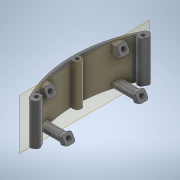
# Autodesk Inventor part: side_prot_stab
Saved by Autodesk Inventor 2020 (Build 240168000, 168)
## iProperties
Created: 2023-12-20
Part Number: side_prot_stab
Material: Пластик АБС
Document SubType Name: Modeling
Designer: denis
Density: 1.06 g/cm^3
Appearance: Гладкая — черная
Author: denis
Autodesk Inventor part; units mm, degrees
(part 1 of 3)
ref_plane "XZ Plane" through (0, 0, 0) normal (0, 1, 0) x (-1, 0, 0)
sketch "Эскиз1" plane through (0, 0, 0) normal (0, 1, 0) x (-1, 0, 0)
  arc A0 (93.050296, -48.648149) -> (93.050296, 48.648149) centre (0, 0) ccw
  line L0 (0, 0) -> (0, -105) construction
  line L1 (0, 0) -> (105, 0) construction
  line L2 (0, 0) -> (74.246212, -74.246212) construction
  line L3 (0, 0) -> (105, 0) construction
  arc A1 (47.06678, -85.957653) -> (85.957653, -47.06678) centre (0, 0) ccw construction
  line L4 (0, 0) -> (-74.246212, -74.246212) construction
  line L5 (73.892659, -46.315494) -> (46.315494, -73.892659)
  line L6 (76.013979, -34.294679) -> (34.294679, -76.013979)
  circle A2 centre (37.830213, -79.549513) radius 1.6
  circle A3 centre (79.549513, -37.830213) radius 1.6
  line L7 (37.830213, -79.549513) -> (79.549513, -37.830213) construction
  line L8 (87.179537, -38.389169) -> (83.085047, -34.294679)
  line L9 (38.389169, -87.179537) -> (34.294679, -83.085047)
  line L10 (88.270396, -49.379523) -> (85.206367, -46.315494)
  line L11 (49.379523, -88.270396) -> (46.315494, -85.206367)
  arc A4 (74.246212, -74.246212) -> (91.09999, -52.209117) centre (0, 0) ccw construction
  arc A5 (52.209117, -91.09999) -> (74.246212, -74.246212) centre (0, 0) ccw construction
  arc A6 (48.648149, -93.050296) -> (49.379523, -88.270396) centre (47.258202, -90.391716) ccw
  arc A7 (88.270396, -49.379523) -> (93.050296, -48.648149) centre (90.391716, -47.258202) ccw
  arc A8 (46.315494, -73.892659) -> (46.315494, -85.206367) centre (51.972348, -79.549513) ccw
  arc A9 (85.206367, -46.315494) -> (73.892659, -46.315494) centre (79.549513, -51.972348) ccw
  arc A10 (34.294679, -76.013979) -> (34.294679, -83.085047) centre (37.830213, -79.549513) ccw
  arc A11 (83.085047, -34.294679) -> (76.013979, -34.294679) centre (79.549513, -37.830213) ccw
  arc A12 (40.465243, -89.255611) -> (47.06678, -85.957653) centre (0, 0) ccw construction
  arc A13 (85.957653, -47.06678) -> (89.255611, -40.465243) centre (0, 0) ccw construction
  arc A14 (90.439454, -37.745267) -> (90.439454, 37.745267) centre (0, 0) ccw
  arc A15 (87.179537, -38.389169) -> (90.439454, -37.745267) centre (88.593751, -36.974956) ccw
  arc A16 (37.745267, -90.439454) -> (38.389169, -87.179537) centre (36.974956, -88.593751) ccw
  arc A17 (38.389169, 87.179537) -> (37.745267, 90.439454) centre (36.974956, 88.593751) ccw construction
  arc A18 (49.379523, 88.270396) -> (48.648149, 93.050296) centre (47.258202, 90.391716) ccw
  line L12 (49.379523, 88.270396) -> (46.315494, 85.206367)
  arc A19 (46.315494, 85.206367) -> (46.315494, 73.892659) centre (51.972348, 79.549513) ccw
  line L13 (38.389169, 87.179537) -> (34.294679, 83.085047) construction
  arc A20 (34.294679, 83.085047) -> (34.294679, 76.013979) centre (37.830213, 79.549513) ccw construction
  line L14 (34.294679, 76.013979) -> (76.013979, 34.294679) construction
  line L15 (46.315494, 73.892659) -> (73.892659, 46.315494)
  arc A21 (76.013979, 34.294679) -> (83.085047, 34.294679) centre (79.549513, 37.830213) ccw
  circle A22 centre (37.830213, 79.549513) radius 1.6
  circle A23 centre (79.549513, 37.830213) radius 1.6
  line L16 (87.179537, 38.389169) -> (83.085047, 34.294679)
  arc A24 (90.439454, 37.745267) -> (87.179537, 38.389169) centre (88.593751, 36.974956) ccw
  arc A25 (93.050296, 48.648149) -> (88.270396, 49.379523) centre (90.391716, 47.258202) ccw
  line L17 (88.270396, 49.379523) -> (85.206367, 46.315494)
  arc A26 (73.892659, 46.315494) -> (85.206367, 46.315494) centre (79.549513, 51.972348) ccw
  arc A27 (-87.179537, 38.389169) -> (-90.439454, 37.745267) centre (-88.593751, 36.974956) ccw
  arc A28 (-88.270396, 49.379523) -> (-93.050296, 48.648149) centre (-90.391716, 47.258202) ccw
  line L18 (-88.270396, 49.379523) -> (-85.206367, 46.315494)
  arc A29 (-85.206367, 46.315494) -> (-73.892659, 46.315494) centre (-79.549513, 51.972348) ccw
  line L19 (-87.179537, 38.389169) -> (-83.085047, 34.294679)
  arc A30 (-83.085047, 34.294679) -> (-76.013979, 34.294679) centre (-79.549513, 37.830213) ccw
  line L20 (-76.013979, 34.294679) -> (-34.294679, 76.013979) construction
  line L21 (-73.892659, 46.315494) -> (-46.315494, 73.892659)
  arc A31 (-34.294679, 76.013979) -> (-34.294679, 83.085047) centre (-37.830213, 79.549513) ccw construction
  circle A32 centre (-79.549513, 37.830213) radius 1.6
  circle A33 centre (-37.830213, 79.549513) radius 1.6
  line L22 (-38.389169, 87.179537) -> (-34.294679, 83.085047) construction
  arc A34 (-37.745267, 90.439454) -> (-38.389169, 87.179537) centre (-36.974956, 88.593751) ccw construction
  arc A35 (-48.648149, 93.050296) -> (-49.379523, 88.270396) centre (-47.258202, 90.391716) ccw
  line L23 (-49.379523, 88.270396) -> (-46.315494, 85.206367)
  arc A36 (-46.315494, 73.892659) -> (-46.315494, 85.206367) centre (-51.972348, 79.549513) ccw
  arc A37 (-38.389169, -87.179537) -> (-37.745267, -90.439454) centre (-36.974956, -88.593751) ccw
  arc A38 (-49.379523, -88.270396) -> (-48.648149, -93.050296) centre (-47.258202, -90.391716) ccw
  line L24 (-49.379523, -88.270396) -> (-46.315494, -85.206367)
  arc A39 (-46.315494, -85.206367) -> (-46.315494, -73.892659) centre (-51.972348, -79.549513) ccw
  line L25 (-38.389169, -87.179537) -> (-34.294679, -83.085047)
  arc A40 (-34.294679, -83.085047) -> (-34.294679, -76.013979) centre (-37.830213, -79.549513) ccw
  line L26 (-34.294679, -76.013979) -> (-76.013979, -34.294679)
  line L27 (-46.315494, -73.892659) -> (-73.892659, -46.315494)
  arc A41 (-76.013979, -34.294679) -> (-83.085047, -34.294679) centre (-79.549513, -37.830213) ccw
  circle A42 centre (-37.830213, -79.549513) radius 1.6
  circle A43 centre (-79.549513, -37.830213) radius 1.6
  line L28 (-87.179537, -38.389169) -> (-83.085047, -34.294679)
  arc A44 (-90.439454, -37.745267) -> (-87.179537, -38.389169) centre (-88.593751, -36.974956) ccw
  arc A45 (-93.050296, -48.648149) -> (-88.270396, -49.379523) centre (-90.391716, -47.258202) ccw
  line L29 (-88.270396, -49.379523) -> (-85.206367, -46.315494)
  arc A46 (-73.892659, -46.315494) -> (-85.206367, -46.315494) centre (-79.549513, -51.972348) ccw
  arc A47 (0, 67.941027) -> (23.782532, 76.596871) centre (0, 104.941027) ccw construction
  arc A48 (-23.782532, 76.596871) -> (0, 67.941027) centre (0, 104.941027) ccw construction
  line L30 (-23.782532, 76.596871) -> (-29.181616, 81.127042) construction
  arc A49 (-28.545172, 71.457103) -> (5.541335, 61.291358) centre (0, 104.941027) ccw construction
  arc A50 (5.541335, 61.291358) -> (28.545172, 71.457103) centre (0, 104.941027) ccw construction
  line L31 (23.782532, 76.596871) -> (26.803217, 79.131416) construction
  line L32 (-34.149097, 76.159561) -> (-28.545172, 71.457103) construction
  line L33 (31.223246, 73.704372) -> (28.545172, 71.457103) construction
  line L34 (26.803217, 79.131416) -> (23.782532, 76.596871) construction
  line L35 (30.759145, 79.549513) -> (31.448305, 78.860353) construction
  line L36 (31.223246, 73.704372) -> (28.545172, 71.457103) construction
  line L37 (-28.545172, 71.457103) -> (-34.149097, 76.159561) construction
  line L38 (-23.782532, 76.596871) -> (-29.181616, 81.127042) construction
  line L39 (-29.181616, 81.127042) -> (-34.149097, 76.159561) construction
  arc A51 (31.223246, 73.704372) -> (26.646177, 78.99965) centre (28.973431, 76.385479) ccw construction
  arc A52 (-26.646177, 78.99965) -> (-31.223246, 73.704372) centre (-28.973431, 76.385479) ccw construction
  arc A53 (-24.841986, 61.889251) -> (-25.418693, 62.824241) centre (-28.115423, 60.51553) ccw
  line L40 (-24.841986, 61.889251) -> (-23.83128, 59.480842)
  line L41 (-43.035533, 94.165467) -> (-18.380184, 65.366371)
  arc A54 (-0.616138, 59.304458) -> (0.616138, 59.304458) centre (0, 61.207186) ccw
  line L42 (-2.671978, 59.970176) -> (-4.5, 60.562123) construction
  arc A55 (-2.515557, 60.080545) -> (-2.671978, 59.970176) centre (0, 56.349329) ccw construction
  line L43 (-15.158499, 56.590699) -> (-21.004883, 57.332824)
  arc A56 (-14.511894, 56.446301) -> (-15.158499, 56.590699) centre (-15.605539, 53.068959) ccw
  line L44 (-17.477038, 64.764325) -> (-0.616138, 59.304458)
  line L45 (-14.511894, 56.446301) -> (-0.616138, 51.946601)
  arc A57 (44.027132, 95.32372) -> (43.576979, 95.530345) centre (0, 0) ccw construction
  circle A58 centre (20.557843, 60.854564) radius 1.55
  arc A59 (-34.190883, 73.070746) -> (-37.124381, 73.184277) centre (-35.710168, 71.770063) ccw
  line L46 (-34.190883, 73.070746) -> (-27.055798, 64.736489) construction
  line L47 (-25.418693, 62.824241) -> (-34.190883, 73.070746)
  arc A60 (-23.83128, 59.480842) -> (-21.004883, 57.332824) centre (-20.557843, 60.854564) ccw
  arc A61 (-18.380184, 65.366371) -> (-17.477038, 64.764325) centre (-16.8609, 66.667053) ccw
  circle A62 centre (-20.557843, 60.854564) radius 1.55
  arc A63 (15.158499, 56.590699) -> (14.511894, 56.446301) centre (15.605539, 53.068959) ccw
  line L48 (15.158499, 56.590699) -> (21.004883, 57.332824)
  arc A64 (25.418693, 62.824241) -> (24.841986, 61.889251) centre (28.115423, 60.51553) ccw
  line L49 (24.841986, 61.889251) -> (23.83128, 59.480842)
  arc A65 (21.004883, 57.332824) -> (23.83128, 59.480842) centre (20.557843, 60.854564) ccw
  line L50 (25.418693, 62.824241) -> (34.190883, 73.070746)
  arc A66 (37.124381, 73.184277) -> (34.190883, 73.070746) centre (35.710168, 71.770063) ccw
  line L51 (14.511894, 56.446301) -> (0.616138, 51.946601)
  arc A67 (17.477038, 64.764325) -> (18.380184, 65.366371) centre (16.8609, 66.667053) ccw
  line L52 (17.477038, 64.764325) -> (0.616138, 59.304458)
  line L53 (-37.124381, 73.184277) -> (-76.013979, 34.294679)
  line L54 (37.124381, 73.184277) -> (76.013979, 34.294679)
  arc A68 (-45.41996, 94.667984) -> (-48.648149, 93.050296) centre (0, 0) ccw
  arc A69 (-43.035533, 94.165467) -> (-45.41996, 94.667984) centre (-44.554817, 92.864785) ccw
  arc A70 (-0.616138, 51.946601) -> (0.616138, 51.946601) centre (0, 53.849329) ccw
  arc A71 (-48.648149, 93.050296) -> (-93.050296, 48.648149) centre (0, 0) ccw construction
  line L55 (43.035533, 94.165467) -> (18.380184, 65.366371)
  arc A72 (48.648149, 93.050296) -> (45.41996, 94.667984) centre (0, 0) ccw
  arc A73 (45.41996, 94.667984) -> (43.035533, 94.165467) centre (44.554817, 92.864785) ccw
  arc A74 (93.050296, 48.648149) -> (-44.027132, 95.32372) centre (0, 0) ccw construction
  arc A75 (-93.050296, -48.648149) -> (-48.648149, -93.050296) centre (0, 0) ccw construction
  arc A76 (-93.050296, 48.648149) -> (-93.050296, -48.648149) centre (0, 0) ccw
  arc A77 (-90.439454, -37.745267) -> (-37.745267, -90.439454) centre (0, 0) ccw construction
  arc A78 (-90.439454, 37.745267) -> (-90.439454, -37.745267) centre (0, 0) ccw
  arc A79 (90.439454, 37.745267) -> (-90.439454, 37.745267) centre (0, 0) ccw construction
  arc A80 (-37.745267, -90.439454) -> (37.745267, -90.439454) centre (0, 0) ccw
  arc A81 (-48.648149, -93.050296) -> (48.648149, -93.050296) centre (0, 0) ccw
  circle A82 centre (0, 55.599329) radius 1.75
  point P0 (60.104076, -60.104076)
  point P1 (55.154329, -55.154329)
  point P2 (78.135299, -39.244426)
  point P3 (39.244426, -78.135299)
  point P4 (52.209117, 91.09999)
  point P5 (39.244426, 78.135299)
  point P6 (47.06678, 85.957653)
  point P7 (55.154329, 55.154329)
  point P8 (60.104076, 60.104076)
  point P9 (91.09999, 52.209117)
  point P10 (78.135299, 39.244426)
  point P11 (85.957653, 47.06678)
  point P12 (-91.09999, 52.209117)
  point P13 (-78.135299, 39.244426)
  point P14 (-85.957653, 47.06678)
  point P15 (-55.154329, 55.154329)
  point P16 (-60.104076, 60.104076)
  point P17 (-52.209117, 91.09999)
  point P18 (-39.244426, 78.135299)
  point P19 (-47.06678, 85.957653)
  point P20 (-52.209117, -91.09999)
  point P21 (-39.244426, -78.135299)
  point P22 (-47.06678, -85.957653)
  point P23 (-55.154329, -55.154329)
  point P24 (-60.104076, -60.104076)
  point P25 (-91.09999, -52.209117)
  point P26 (-78.135299, -39.244426)
  point P27 (-85.957653, -47.06678)
  point P28 (-28.545172, 71.457103)
  point P29 (-39.282973, 89.782226)
  point P30 (0, 95.32372)
  point P31 (0, 66.207186)
  point P32 (-44.027132, 95.32372)
  point P33 (0, 59.207186)
  point P34 (44.554817, 92.864785)
  point P35 (-42.426407, 67.882251)
  point P36 (-22.705861, 58.028168)
  point P37 (-21.49571, 59.620504)
  dimension "d1" = 45
  dimension "d3" = 7
  dimension "d5" = 20
  dimension "d9" = 7
  dimension "d10" = 3.2
  dimension "d14" = 59
  dimension "d15" = 83
  dimension "d17" = 69
  dimension "d19" = 55
  dimension "d20" = 3
  dimension "d21" = 8
  dimension "d22" = 5
  dimension "d23" = 2
  dimension "d26" = 360
  dimension "d39" = 7
  dimension "d44" = 120
  dimension "d45" = 3.55
  dimension "d46" = 2
  dimension "d47" = 2.61189
  dimension "d48" = 2
  dimension "d49" = 105
  dimension "d50" = 2
  dimension "d54" = 3.5
  dimension "d55" = 2
  constraints: 165 point on circle, 112 end point, 83 centre point, 38 point on line, 27 tangent, 23 symmetric about line, 8 midpoint, 6 equal radius, 4 coincident, 4 collinear, 4 parallel, 3 horizontal, 2 vertical, 1 equal length, 1 perpendicular, 234 other
  measures "d1" angle of L2 L3
  measures "d3" radial gap between concentric circles of A0 A1
  measures "d5" distance from line of L5 L2.end
  measures "d9" distance between parallel lines of L5 L6
  measures "d10" diameter of A2
  measures "d14" distance of L7.end L7.start
  measures "d15" distance from line of point (0, 0) L7
  measures "d17" distance between parallel lines of L8 L9
  measures "d19" distance between parallel lines of L11 L10
  measures "d20" radius of A6
  measures "d21" radius of A8
  measures "d22" radius of A10
  measures "d23" radius of A15
  measures "d39" distance of point (0, 66.207) point (0, 59.207)
  measures "d44" angle of L40 L43
  measures "d45" radius of A53
  measures "d46" distance of point (-22.706, 58.028) point (-21.496, 59.621)
  measures "d47" distance of L40.start L40.end
  measures "d48" radius of A69
  measures "d49" radius of A68
  measures "d50" radius of A70
  measures "d54" diameter of A82
extrude "outer" add sketch "Эскиз1" along normal blind 2 contours A7 L10 A9 L5 A8 L11 A6 A81 A38 L24 A39 L27 A46 L29 A45 A76 A28 L18 A29 L21 A36 L23 A35 A68 A69 L41 A61 L44 A54 L52 A67 L55 A73 A72 A18 L12 A19 L15 A26 L17 A25 A0 | A82
sketch "Эскиз2" plane through (0, 2, 0) normal (0, 1, 0) x (1, 0, 0)
  arc A0 (-46.315494, -85.206367) -> (-46.315494, -73.892659) centre (-51.972348, -79.549513) ccw construction
  line L0 (-46.315494, -85.206367) -> (-49.379523, -88.270396) construction
  arc A1 (-49.379523, -88.270396) -> (-48.648149, -93.050296) centre (-47.258202, -90.391716) ccw construction
  arc A2 (-48.648149, -93.050296) -> (-45.41996, -94.667984) centre (0, 0) ccw construction
  arc A3 (-45.41996, -94.667984) -> (-43.035533, -94.165467) centre (-44.554817, -92.864785) ccw construction
  line L1 (-43.035533, -94.165467) -> (-18.380184, -65.366371) construction
  arc A4 (-17.477038, -64.764325) -> (-18.380184, -65.366371) centre (-16.8609, -66.667053) ccw construction
  line L2 (-17.477038, -64.764325) -> (-0.616138, -59.304458) construction
  arc A5 (0.616138, -59.304458) -> (-0.616138, -59.304458) centre (0, -61.207186) ccw construction
  line L3 (0.616138, -59.304458) -> (17.477038, -64.764325) construction
  arc A6 (18.380184, -65.366371) -> (17.477038, -64.764325) centre (16.8609, -66.667053) ccw construction
  line L4 (18.380184, -65.366371) -> (43.035533, -94.165467) construction
  arc A7 (43.035533, -94.165467) -> (45.41996, -94.667984) centre (44.554817, -92.864785) ccw construction
  arc A8 (45.41996, -94.667984) -> (48.648149, -93.050296) centre (0, 0) ccw construction
  arc A9 (48.648149, -93.050296) -> (49.379523, -88.270396) centre (47.258202, -90.391716) ccw construction
  line L5 (49.379523, -88.270396) -> (46.315494, -85.206367) construction
  arc A10 (46.315494, -73.892659) -> (46.315494, -85.206367) centre (51.972348, -79.549513) ccw construction
  line L6 (46.315494, -73.892659) -> (73.892659, -46.315494) construction
  arc A11 (85.206367, -46.315494) -> (73.892659, -46.315494) centre (79.549513, -51.972348) ccw construction
  line L7 (85.206367, -46.315494) -> (88.270396, -49.379523) construction
  arc A12 (88.270396, -49.379523) -> (93.050296, -48.648149) centre (90.391716, -47.258202) ccw construction
  arc A13 (93.050296, -48.648149) -> (93.050296, 48.648149) centre (0, 0) ccw construction
  arc A14 (93.050296, 48.648149) -> (88.270396, 49.379523) centre (90.391716, 47.258202) ccw construction
  line L8 (88.270396, 49.379523) -> (85.206367, 46.315494) construction
  arc A15 (73.892659, 46.315494) -> (85.206367, 46.315494) centre (79.549513, 51.972348) ccw construction
  line L9 (73.892659, 46.315494) -> (46.315494, 73.892659) construction
  arc A16 (46.315494, 85.206367) -> (46.315494, 73.892659) centre (51.972348, 79.549513) ccw construction
  line L10 (46.315494, 85.206367) -> (49.379523, 88.270396) construction
  arc A17 (49.379523, 88.270396) -> (48.648149, 93.050296) centre (47.258202, 90.391716) ccw construction
  arc A18 (48.648149, 93.050296) -> (-48.648149, 93.050296) centre (0, 0) ccw construction
  arc A19 (-48.648149, 93.050296) -> (-49.379523, 88.270396) centre (-47.258202, 90.391716) ccw construction
  line L11 (-49.379523, 88.270396) -> (-46.315494, 85.206367) construction
  arc A20 (-46.315494, 73.892659) -> (-46.315494, 85.206367) centre (-51.972348, 79.549513) ccw construction
  line L12 (-46.315494, 73.892659) -> (-73.892659, 46.315494) construction
  arc A21 (-85.206367, 46.315494) -> (-73.892659, 46.315494) centre (-79.549513, 51.972348) ccw construction
  line L13 (-85.206367, 46.315494) -> (-88.270396, 49.379523) construction
  arc A22 (-88.270396, 49.379523) -> (-93.050296, 48.648149) centre (-90.391716, 47.258202) ccw construction
  arc A23 (-93.050296, 48.648149) -> (-93.050296, -48.648149) centre (0, 0) ccw construction
  arc A24 (-93.050296, -48.648149) -> (-88.270396, -49.379523) centre (-90.391716, -47.258202) ccw construction
  line L14 (-88.270396, -49.379523) -> (-85.206367, -46.315494) construction
  arc A25 (-73.892659, -46.315494) -> (-85.206367, -46.315494) centre (-79.549513, -51.972348) ccw construction
  line L15 (-73.892659, -46.315494) -> (-46.315494, -73.892659) construction
  circle A26 centre (-37.830213, 79.549513) radius 1.6 construction
  circle A27 centre (-79.549513, 37.830213) radius 1.6 construction
  circle A28 centre (-79.549513, -37.830213) radius 1.6 construction
  circle A29 centre (79.549513, -37.830213) radius 1.6 construction
  circle A30 centre (37.830213, 79.549513) radius 1.6 construction
  circle A31 centre (79.549513, 37.830213) radius 1.6 construction
  circle A32 centre (-20.557843, -60.854564) radius 1.55 construction
  circle A33 centre (20.557843, -60.854564) radius 1.55 construction
  circle A34 centre (37.830213, -79.549513) radius 1.6 construction
  circle A35 centre (-37.830213, -79.549513) radius 1.6 construction
  line L16 (-83.085047, -34.294679) -> (-87.179537, -38.389169) construction
  arc A36 (-90.439454, -37.745267) -> (-87.179537, -38.389169) centre (-88.593751, -36.974956) ccw construction
  arc A37 (-90.439454, 37.745267) -> (-90.439454, -37.745267) centre (0, 0) ccw construction
  arc A38 (-87.179537, 38.389169) -> (-90.439454, 37.745267) centre (-88.593751, 36.974956) ccw construction
  line L17 (-87.179537, 38.389169) -> (-83.085047, 34.294679) construction
  arc A39 (-83.085047, 34.294679) -> (-76.013979, 34.294679) centre (-79.549513, 37.830213) ccw construction
  line L18 (-76.013979, 34.294679) -> (-34.294679, 76.013979) construction
  arc A40 (-34.294679, 76.013979) -> (-34.294679, 83.085047) centre (-37.830213, 79.549513) ccw construction
  line L19 (-34.294679, 83.085047) -> (-38.389169, 87.179537) construction
  arc A41 (-37.745267, 90.439454) -> (-38.389169, 87.179537) centre (-36.974956, 88.593751) ccw construction
  arc A42 (37.745267, 90.439454) -> (-37.745267, 90.439454) centre (0, 0) ccw construction
  arc A43 (38.389169, 87.179537) -> (37.745267, 90.439454) centre (36.974956, 88.593751) ccw construction
  line L20 (38.389169, 87.179537) -> (34.294679, 83.085047) construction
  arc A44 (34.294679, 83.085047) -> (34.294679, 76.013979) centre (37.830213, 79.549513) ccw construction
  line L21 (34.294679, 76.013979) -> (76.013979, 34.294679) construction
  arc A45 (76.013979, 34.294679) -> (83.085047, 34.294679) centre (79.549513, 37.830213) ccw construction
  line L22 (83.085047, 34.294679) -> (87.179537, 38.389169) construction
  arc A46 (90.439454, 37.745267) -> (87.179537, 38.389169) centre (88.593751, 36.974956) ccw construction
  arc A47 (90.439454, -37.745267) -> (90.439454, 37.745267) centre (0, 0) ccw construction
  arc A48 (87.179537, -38.389169) -> (90.439454, -37.745267) centre (88.593751, -36.974956) ccw construction
  line L23 (87.179537, -38.389169) -> (83.085047, -34.294679) construction
  arc A49 (83.085047, -34.294679) -> (76.013979, -34.294679) centre (79.549513, -37.830213) ccw construction
  line L24 (76.013979, -34.294679) -> (37.124381, -73.184277) construction
  arc A50 (34.190883, -73.070746) -> (37.124381, -73.184277) centre (35.710168, -71.770063) ccw construction
  line L25 (34.190883, -73.070746) -> (25.418693, -62.824241) construction
  arc A51 (24.841986, -61.889251) -> (25.418693, -62.824241) centre (28.115423, -60.51553) ccw construction
  line L26 (24.841986, -61.889251) -> (23.83128, -59.480842) construction
  arc A52 (23.83128, -59.480842) -> (21.004883, -57.332824) centre (20.557843, -60.854564) ccw construction
  line L27 (21.004883, -57.332824) -> (15.158499, -56.590699) construction
  arc A53 (14.511894, -56.446301) -> (15.158499, -56.590699) centre (15.605539, -53.068959) ccw construction
  line L28 (14.511894, -56.446301) -> (0.616138, -51.946601) construction
  arc A54 (0.616138, -51.946601) -> (-0.616138, -51.946601) centre (0, -53.849329) ccw construction
  line L29 (-0.616138, -51.946601) -> (-14.511894, -56.446301) construction
  arc A55 (-15.158499, -56.590699) -> (-14.511894, -56.446301) centre (-15.605539, -53.068959) ccw construction
  line L30 (-15.158499, -56.590699) -> (-21.004883, -57.332824) construction
  arc A56 (-21.004883, -57.332824) -> (-23.83128, -59.480842) centre (-20.557843, -60.854564) ccw construction
  line L31 (-23.83128, -59.480842) -> (-24.841986, -61.889251) construction
  arc A57 (-25.418693, -62.824241) -> (-24.841986, -61.889251) centre (-28.115423, -60.51553) ccw construction
  line L32 (-25.418693, -62.824241) -> (-34.190883, -73.070746) construction
  arc A58 (-37.124381, -73.184277) -> (-34.190883, -73.070746) centre (-35.710168, -71.770063) ccw construction
  line L33 (-37.124381, -73.184277) -> (-76.013979, -34.294679) construction
  arc A59 (-76.013979, -34.294679) -> (-83.085047, -34.294679) centre (-79.549513, -37.830213) ccw construction
  line L34 (0, 0) -> (-74.246212, 74.246212) construction
  line L35 (0, 0) -> (-105, 0) construction
  line L36 (0, 0) -> (0, 105) construction
  line L37 (0, 0) -> (74.246212, 74.246212) construction
  line L38 (-46.669048, 63.63961) -> (-26.870058, 43.84062)
  line L39 (-63.63961, 46.669048) -> (-43.84062, 26.870058)
  line L40 (-67.882251, 42.426407) -> (-43.133514, 17.67767) construction
  line L41 (-41.012193, 26.870058) -> (-26.870058, 41.012193)
  line L42 (-43.134692, 17.676491) -> (-17.67767, 43.133514) construction
  circle A60 centre (-21.92031, 43.133514) radius 1.6
  circle A61 centre (-43.133514, 21.92031) radius 1.6
  line L43 (-33.941125, 33.941125) -> (-30.405592, 30.405592) construction
  arc A62 (-26.870058, 41.012193) -> (-26.870058, 43.84062) centre (-28.284271, 42.426407) ccw
  arc A63 (-43.84062, 26.870058) -> (-41.012193, 26.870058) centre (-42.426407, 28.284271) ccw
  line L44 (-67.882251, 42.426407) -> (-42.426407, 67.882251)
  line L45 (-43.133514, 21.92031) -> (-21.92031, 43.133514) construction
  line L46 (-63.63961, -46.669048) -> (-43.84062, -26.870058)
  line L47 (-42.426407, -67.882251) -> (-67.882251, -42.426407)
  line L48 (-46.669048, -63.63961) -> (-26.870058, -43.84062)
  line L49 (-26.870058, -41.012193) -> (-41.012193, -26.870058)
  arc A64 (-41.012193, -26.870058) -> (-43.84062, -26.870058) centre (-42.426407, -28.284271) ccw
  circle A65 centre (-43.133514, -21.92031) radius 1.6
  circle A66 centre (-21.92031, -43.133514) radius 1.6
  arc A67 (-26.870058, -43.84062) -> (-26.870058, -41.012193) centre (-28.284271, -42.426407) ccw
  line L50 (46.669048, -63.63961) -> (26.870058, -43.84062)
  line L51 (67.882251, -42.426407) -> (42.426407, -67.882251)
  line L52 (63.63961, -46.669048) -> (43.84062, -26.870058)
  line L53 (41.012193, -26.870058) -> (26.870058, -41.012193)
  arc A68 (26.870058, -41.012193) -> (26.870058, -43.84062) centre (28.284271, -42.426407) ccw
  circle A69 centre (21.92031, -43.133514) radius 1.6
  circle A70 centre (43.133514, -21.92031) radius 1.6
  arc A71 (43.84062, -26.870058) -> (41.012193, -26.870058) centre (42.426407, -28.284271) ccw
  line L54 (63.63961, 46.669048) -> (43.84062, 26.870058)
  line L55 (42.426407, 67.882251) -> (67.882251, 42.426407)
  line L56 (46.669048, 63.63961) -> (26.870058, 43.84062)
  line L57 (26.870058, 41.012193) -> (41.012193, 26.870058)
  arc A72 (41.012193, 26.870058) -> (43.84062, 26.870058) centre (42.426407, 28.284271) ccw
  circle A73 centre (43.133514, 21.92031) radius 1.6
  circle A74 centre (21.92031, 43.133514) radius 1.6
  arc A75 (26.870058, 43.84062) -> (26.870058, 41.012193) centre (28.284271, 42.426407) ccw
  line L58 (-21.92031, 43.133514) -> (21.92031, 43.133514) construction
  line L59 (-20.67767, 40.133514) -> (20.67767, 40.133514) construction
  line L60 (-20.67767, 46.133514) -> (20.67767, 46.133514) construction
  line L61 (42.426407, 67.882251) -> (14.225288, 39.681132) construction
  line L62 (67.882251, 42.426407) -> (40.318778, 14.862934) construction
  line L63 (43.134692, 17.676491) -> (16.615831, 44.195352) construction
  arc A76 (-21.669819, 47.125663) -> (-21.669819, 39.141365) centre (-21.92031, 43.133514) ccw construction
  line L64 (-42.426407, 67.882251) -> (-21.669819, 47.125663)
  arc A77 (-19.274559, 46.133514) -> (-21.669819, 47.125663) centre (-21.92031, 43.133514) ccw
  arc A78 (-21.669819, 39.141365) -> (-19.274559, 40.133514) centre (-21.92031, 43.133514) ccw
  arc A79 (-19.274559, 40.133514) -> (-19.274559, 46.133514) centre (-21.92031, 43.133514) ccw construction
  line L65 (-21.669819, 47.125663) -> (-17.67767, 43.133514) construction
  line L66 (-19.274559, 46.133514) -> (0, 46.133514)
  line L67 (-30.405592, 30.405592) -> (-21.669819, 39.141365)
  line L68 (-67.882251, 42.426407) -> (-47.125663, 21.669819)
  arc A80 (-47.125663, 21.669819) -> (-46.133514, 19.274559) centre (-43.133514, 21.92031) ccw
  arc A81 (-40.133514, 19.274559) -> (-39.141365, 21.669819) centre (-43.133514, 21.92031) ccw
  line L69 (-46.133514, 19.274559) -> (-46.133514, 0)
  line L70 (-30.405592, 30.405592) -> (-39.141365, 21.669819)
  line L71 (-19.274559, 40.133514) -> (0, 40.133514)
  line L72 (-40.133514, 19.274559) -> (-40.133514, 0)
  line L73 (-40.133514, -19.274559) -> (-40.133514, 0)
  line L74 (-46.133514, -19.274559) -> (-46.133514, 0)
  arc A82 (-46.133514, -19.274559) -> (-47.125663, -21.669819) centre (-43.133514, -21.92031) ccw
  line L75 (-67.882251, -42.426407) -> (-47.125663, -21.669819)
  arc A83 (-39.141365, -21.669819) -> (-40.133514, -19.274559) centre (-43.133514, -21.92031) ccw
  line L76 (-30.405592, -30.405592) -> (-39.141365, -21.669819)
  line L77 (-30.405592, -30.405592) -> (-21.669819, -39.141365)
  arc A84 (-19.274559, -40.133514) -> (-21.669819, -39.141365) centre (-21.92031, -43.133514) ccw
  line L78 (-19.274559, -40.133514) -> (0, -40.133514)
  line L79 (-19.274559, -46.133514) -> (0, -46.133514)
  arc A85 (-21.669819, -47.125663) -> (-19.274559, -46.133514) centre (-21.92031, -43.133514) ccw
  line L80 (-42.426407, -67.882251) -> (-21.669819, -47.125663)
  line L81 (19.274559, -40.133514) -> (0, -40.133514)
  line L82 (19.274559, -46.133514) -> (0, -46.133514)
  arc A86 (19.274559, -46.133514) -> (21.669819, -47.125663) centre (21.92031, -43.133514) ccw
  line L83 (42.426407, -67.882251) -> (21.669819, -47.125663)
  arc A87 (21.669819, -39.141365) -> (19.274559, -40.133514) centre (21.92031, -43.133514) ccw
  line L84 (30.405592, -30.405592) -> (21.669819, -39.141365)
  line L85 (30.405592, -30.405592) -> (39.141365, -21.669819)
  arc A88 (40.133514, -19.274559) -> (39.141365, -21.669819) centre (43.133514, -21.92031) ccw
  line L86 (40.133514, -19.274559) -> (40.133514, 0)
  line L87 (46.133514, -19.274559) -> (46.133514, 0)
  arc A89 (47.125663, -21.669819) -> (46.133514, -19.274559) centre (43.133514, -21.92031) ccw
  line L88 (67.882251, -42.426407) -> (47.125663, -21.669819)
  line L89 (40.133514, 19.274559) -> (40.133514, 0)
  line L90 (46.133514, 19.274559) -> (46.133514, 0)
  arc A90 (46.133514, 19.274559) -> (47.125663, 21.669819) centre (43.133514, 21.92031) ccw
  line L91 (67.882251, 42.426407) -> (47.125663, 21.669819)
  arc A91 (39.141365, 21.669819) -> (40.133514, 19.274559) centre (43.133514, 21.92031) ccw
  line L92 (30.405592, 30.405592) -> (39.141365, 21.669819)
  line L93 (30.405592, 30.405592) -> (21.669819, 39.141365)
  arc A92 (19.274559, 40.133514) -> (21.669819, 39.141365) centre (21.92031, 43.133514) ccw
  line L94 (19.274559, 40.133514) -> (0, 40.133514)
  line L95 (19.274559, 46.133514) -> (0, 46.133514)
  arc A93 (21.669819, 47.125663) -> (19.274559, 46.133514) centre (21.92031, 43.133514) ccw
  line L96 (42.426407, 67.882251) -> (21.669819, 47.125663)
  point P0 (-25.455844, 42.426407)
  point P1 (-32.173359, 32.173359)
  point P2 (-42.426407, -25.455844)
  point P3 (-33.941125, -33.941125)
  point P4 (25.455844, -42.426407)
  point P5 (33.941125, -33.941125)
  point P6 (42.426407, 25.455844)
  point P7 (33.941125, 33.941125)
  point P8 (-46.133514, -20.67767)
  point P9 (20.67767, -46.133514)
  point P10 (46.133514, 20.67767)
  point P11 (0, 46.133514)
  point P12 (-46.133514, 0)
  point P13 (0, -46.133514)
  point P14 (46.133514, 0)
  point P15 (0, 40.133514)
  point P16 (40.133514, 0)
  point P17 (0, -40.133514)
  point P18 (-40.133514, 0)
  dimension "d58" = 12
  dimension "d59" = 30
  dimension "d60" = 5
  dimension "d61" = 3.2
  dimension "d62" = 30
  dimension "d63" = 2
  dimension "d64" = 2
  dimension "d65" = 3
  dimension "d68" = 360
  dimension "d70" = 6
  dimension "d71" = 8
  dimension "d74" = 360
  constraints: 118 end point, 52 point on circle, 34 centre point, 28 point on line, 8 symmetric about line, 5 parallel, 4 midpoint, 4 tangent, 1 coincident, 1 collinear, 1 horizontal, 1 perpendicular, 216 other
  measures "d58" distance between parallel lines of L34 L38
  measures "d59" distance between parallel lines of L18 L41
  measures "d60" distance between parallel lines of L41 L42
  measures "d61" diameter of A60
  measures "d62" distance of L45.start L45.end
  measures "d63" radius of A62
  measures "d64" radius of A63
  measures "d65" distance between parallel lines of L42 L45
  measures "d70" distance between parallel lines of L59 L60
  measures "d71" diameter of A76
extrude "inner" add sketch "Эскиз2" against normal blind 2 contours L44 L64 A77 L66 L95 A93 L96 L55 L56 A75 L57 A72 L54 L91 A90 L90 L87 A89 L88 L51 L52 A71 L53 A68 L50 L83 A86 L82 L79 A85 L80 L47 L48 A67 L49 A64 L46 L75 A82 L74 L69 A80 L68 L39 A63 L41 A62 L38
sketch "Эскиз3" plane through (0, 2, 0) normal (0, 1, 0) x (1, 0, 0)
  line L0 (-40.133514, -19.274559) -> (-40.133514, 19.274559) construction
  line L1 (-67.882251, -42.426407) -> (-76.013979, -34.294679) construction
  arc A0 (-76.013979, -34.294679) -> (-83.085047, -34.294679) centre (-79.549513, -37.830213) ccw construction
  line L2 (-83.085047, -34.294679) -> (-87.179537, -38.389169) construction
  arc A1 (-90.439454, -37.745267) -> (-87.179537, -38.389169) centre (-88.593751, -36.974956) ccw construction
  arc A2 (-90.439454, 37.745267) -> (-90.439454, -37.745267) centre (0, 0) ccw construction
  arc A3 (-87.179537, 38.389169) -> (-90.439454, 37.745267) centre (-88.593751, 36.974956) ccw construction
  line L3 (-87.179537, 38.389169) -> (-83.085047, 34.294679) construction
  arc A4 (-83.085047, 34.294679) -> (-76.013979, 34.294679) centre (-79.549513, 37.830213) ccw construction
  line L4 (-76.013979, 34.294679) -> (-67.882251, 42.426407) construction
  line L5 (-67.882251, 42.426407) -> (-47.125663, 21.669819) construction
  arc A5 (-47.125663, 21.669819) -> (-46.133514, 19.274559) centre (-43.133514, 21.92031) ccw construction
  line L6 (-46.133514, 19.274559) -> (-46.133514, -19.274559) construction
  arc A6 (-46.133514, -19.274559) -> (-47.125663, -21.669819) centre (-43.133514, -21.92031) ccw construction
  line L7 (-47.125663, -21.669819) -> (-67.882251, -42.426407) construction
  line L8 (-63.63961, -46.669048) -> (-43.84062, -26.870058) construction
  arc A7 (-41.012193, -26.870058) -> (-43.84062, -26.870058) centre (-42.426407, -28.284271) ccw construction
  line L9 (-41.012193, -26.870058) -> (-26.870058, -41.012193) construction
  arc A8 (-26.870058, -43.84062) -> (-26.870058, -41.012193) centre (-28.284271, -42.426407) ccw construction
  line L10 (-26.870058, -43.84062) -> (-46.669048, -63.63961) construction
  line L11 (-46.669048, -63.63961) -> (-63.63961, -46.669048) construction
  line L12 (-42.426407, -67.882251) -> (-21.669819, -47.125663) construction
  arc A9 (-21.669819, -47.125663) -> (-19.274559, -46.133514) centre (-21.92031, -43.133514) ccw construction
  line L13 (-19.274559, -46.133514) -> (19.274559, -46.133514) construction
  arc A10 (19.274559, -46.133514) -> (21.669819, -47.125663) centre (21.92031, -43.133514) ccw construction
  line L14 (21.669819, -47.125663) -> (42.426407, -67.882251) construction
  line L15 (42.426407, -67.882251) -> (37.124381, -73.184277) construction
  arc A11 (34.190883, -73.070746) -> (37.124381, -73.184277) centre (35.710168, -71.770063) ccw construction
  line L16 (34.190883, -73.070746) -> (25.418693, -62.824241) construction
  arc A12 (24.841986, -61.889251) -> (25.418693, -62.824241) centre (28.115423, -60.51553) ccw construction
  line L17 (24.841986, -61.889251) -> (23.83128, -59.480842) construction
  arc A13 (23.83128, -59.480842) -> (21.004883, -57.332824) centre (20.557843, -60.854564) ccw construction
  line L18 (21.004883, -57.332824) -> (15.158499, -56.590699) construction
  arc A14 (14.511894, -56.446301) -> (15.158499, -56.590699) centre (15.605539, -53.068959) ccw construction
  line L19 (14.511894, -56.446301) -> (0.616138, -51.946601) construction
  arc A15 (0.616138, -51.946601) -> (-0.616138, -51.946601) centre (0, -53.849329) ccw construction
  line L20 (-0.616138, -51.946601) -> (-14.511894, -56.446301) construction
  arc A16 (-15.158499, -56.590699) -> (-14.511894, -56.446301) centre (-15.605539, -53.068959) ccw construction
  line L21 (-15.158499, -56.590699) -> (-21.004883, -57.332824) construction
  arc A17 (-21.004883, -57.332824) -> (-23.83128, -59.480842) centre (-20.557843, -60.854564) ccw construction
  line L22 (-23.83128, -59.480842) -> (-24.841986, -61.889251) construction
  arc A18 (-25.418693, -62.824241) -> (-24.841986, -61.889251) centre (-28.115423, -60.51553) ccw construction
  line L23 (-25.418693, -62.824241) -> (-34.190883, -73.070746) construction
  arc A19 (-37.124381, -73.184277) -> (-34.190883, -73.070746) centre (-35.710168, -71.770063) ccw construction
  line L24 (-37.124381, -73.184277) -> (-42.426407, -67.882251) construction
  line L25 (46.669048, -63.63961) -> (26.870058, -43.84062) construction
  arc A20 (26.870058, -41.012193) -> (26.870058, -43.84062) centre (28.284271, -42.426407) ccw construction
  line L26 (26.870058, -41.012193) -> (41.012193, -26.870058) construction
  arc A21 (43.84062, -26.870058) -> (41.012193, -26.870058) centre (42.426407, -28.284271) ccw construction
  line L27 (43.84062, -26.870058) -> (63.63961, -46.669048) construction
  line L28 (63.63961, -46.669048) -> (46.669048, -63.63961) construction
  line L29 (67.882251, -42.426407) -> (47.125663, -21.669819) construction
  arc A22 (47.125663, -21.669819) -> (46.133514, -19.274559) centre (43.133514, -21.92031) ccw construction
  line L30 (46.133514, -19.274559) -> (46.133514, 19.274559) construction
  arc A23 (46.133514, 19.274559) -> (47.125663, 21.669819) centre (43.133514, 21.92031) ccw construction
  line L31 (47.125663, 21.669819) -> (67.882251, 42.426407) construction
  line L32 (67.882251, 42.426407) -> (76.013979, 34.294679) construction
  arc A24 (76.013979, 34.294679) -> (83.085047, 34.294679) centre (79.549513, 37.830213) ccw construction
  line L33 (83.085047, 34.294679) -> (87.179537, 38.389169) construction
  arc A25 (90.439454, 37.745267) -> (87.179537, 38.389169) centre (88.593751, 36.974956) ccw construction
  arc A26 (90.439454, -37.745267) -> (90.439454, 37.745267) centre (0, 0) ccw construction
  arc A27 (87.179537, -38.389169) -> (90.439454, -37.745267) centre (88.593751, -36.974956) ccw construction
  line L34 (87.179537, -38.389169) -> (83.085047, -34.294679) construction
  arc A28 (83.085047, -34.294679) -> (76.013979, -34.294679) centre (79.549513, -37.830213) ccw construction
  line L35 (76.013979, -34.294679) -> (67.882251, -42.426407) construction
  line L36 (63.63961, 46.669048) -> (43.84062, 26.870058) construction
  arc A29 (41.012193, 26.870058) -> (43.84062, 26.870058) centre (42.426407, 28.284271) ccw construction
  line L37 (41.012193, 26.870058) -> (26.870058, 41.012193) construction
  arc A30 (26.870058, 43.84062) -> (26.870058, 41.012193) centre (28.284271, 42.426407) ccw construction
  line L38 (26.870058, 43.84062) -> (46.669048, 63.63961) construction
  line L39 (46.669048, 63.63961) -> (63.63961, 46.669048) construction
  line L40 (42.426407, 67.882251) -> (21.669819, 47.125663) construction
  arc A31 (21.669819, 47.125663) -> (19.274559, 46.133514) centre (21.92031, 43.133514) ccw construction
  line L41 (19.274559, 46.133514) -> (-19.274559, 46.133514) construction
  arc A32 (-19.274559, 46.133514) -> (-21.669819, 47.125663) centre (-21.92031, 43.133514) ccw construction
  line L42 (-21.669819, 47.125663) -> (-42.426407, 67.882251) construction
  line L43 (-42.426407, 67.882251) -> (-34.294679, 76.013979) construction
  arc A33 (-34.294679, 76.013979) -> (-34.294679, 83.085047) centre (-37.830213, 79.549513) ccw construction
  line L44 (-34.294679, 83.085047) -> (-38.389169, 87.179537) construction
  arc A34 (-37.745267, 90.439454) -> (-38.389169, 87.179537) centre (-36.974956, 88.593751) ccw construction
  arc A35 (37.745267, 90.439454) -> (-37.745267, 90.439454) centre (0, 0) ccw construction
  arc A36 (38.389169, 87.179537) -> (37.745267, 90.439454) centre (36.974956, 88.593751) ccw construction
  line L45 (38.389169, 87.179537) -> (34.294679, 83.085047) construction
  arc A37 (34.294679, 83.085047) -> (34.294679, 76.013979) centre (37.830213, 79.549513) ccw construction
  line L46 (34.294679, 76.013979) -> (42.426407, 67.882251) construction
  line L47 (-19.274559, 40.133514) -> (19.274559, 40.133514) construction
  arc A38 (19.274559, 40.133514) -> (21.669819, 39.141365) centre (21.92031, 43.133514) ccw construction
  line L48 (21.669819, 39.141365) -> (39.141365, 21.669819) construction
  arc A39 (39.141365, 21.669819) -> (40.133514, 19.274559) centre (43.133514, 21.92031) ccw construction
  line L49 (40.133514, 19.274559) -> (40.133514, -19.274559) construction
  arc A40 (40.133514, -19.274559) -> (39.141365, -21.669819) centre (43.133514, -21.92031) ccw construction
  line L50 (39.141365, -21.669819) -> (21.669819, -39.141365) construction
  arc A41 (21.669819, -39.141365) -> (19.274559, -40.133514) centre (21.92031, -43.133514) ccw construction
  line L51 (19.274559, -40.133514) -> (-19.274559, -40.133514) construction
  arc A42 (-19.274559, -40.133514) -> (-21.669819, -39.141365) centre (-21.92031, -43.133514) ccw construction
  line L52 (-21.669819, -39.141365) -> (-39.141365, -21.669819) construction
  arc A43 (-39.141365, -21.669819) -> (-40.133514, -19.274559) centre (-43.133514, -21.92031) ccw construction
  line L53 (-40.133514, -19.274559) -> (-40.133514, 19.274559) construction
  arc A44 (-40.133514, 19.274559) -> (-39.141365, 21.669819) centre (-43.133514, 21.92031) ccw construction
  line L54 (-39.141365, 21.669819) -> (-21.669819, 39.141365) construction
  arc A45 (-21.669819, 39.141365) -> (-19.274559, 40.133514) centre (-21.92031, 43.133514) ccw construction
  circle A46 centre (43.133514, 21.92031) radius 1.6 construction
  circle A47 centre (21.92031, -43.133514) radius 1.6 construction
  circle A48 centre (-21.92031, -43.133514) radius 1.6 construction
  circle A49 centre (-43.133514, -21.92031) radius 1.6 construction
  circle A50 centre (-43.133514, 21.92031) radius 1.6 construction
  circle A51 centre (-21.92031, 43.133514) radius 1.6 construction
  circle A52 centre (43.133514, -21.92031) radius 1.6 construction
  circle A53 centre (21.92031, 43.133514) radius 1.6 construction
  arc A54 (-88.270396, 49.379523) -> (-93.050296, 48.648149) centre (-90.391716, 47.258202) ccw construction
  arc A55 (-93.050296, 48.648149) -> (-93.050296, -48.648149) centre (0, 0) ccw construction
  arc A56 (-93.050296, -48.648149) -> (-88.270396, -49.379523) centre (-90.391716, -47.258202) ccw construction
  line L55 (-88.270396, -49.379523) -> (-85.206367, -46.315494) construction
  arc A57 (-73.892659, -46.315494) -> (-85.206367, -46.315494) centre (-79.549513, -51.972348) ccw construction
  line L56 (-73.892659, -46.315494) -> (-46.315494, -73.892659) construction
  arc A58 (-46.315494, -85.206367) -> (-46.315494, -73.892659) centre (-51.972348, -79.549513) ccw construction
  line L57 (-46.315494, -85.206367) -> (-49.379523, -88.270396) construction
  arc A59 (-49.379523, -88.270396) -> (-48.648149, -93.050296) centre (-47.258202, -90.391716) ccw construction
  arc A60 (-48.648149, -93.050296) -> (-45.41996, -94.667984) centre (0, 0) ccw construction
  arc A61 (-45.41996, -94.667984) -> (-43.035533, -94.165467) centre (-44.554817, -92.864785) ccw construction
  line L58 (-43.035533, -94.165467) -> (-18.380184, -65.366371) construction
  arc A62 (-17.477038, -64.764325) -> (-18.380184, -65.366371) centre (-16.8609, -66.667053) ccw construction
  line L59 (-17.477038, -64.764325) -> (-0.616138, -59.304458) construction
  arc A63 (0.616138, -59.304458) -> (-0.616138, -59.304458) centre (0, -61.207186) ccw construction
  line L60 (0.616138, -59.304458) -> (17.477038, -64.764325) construction
  arc A64 (18.380184, -65.366371) -> (17.477038, -64.764325) centre (16.8609, -66.667053) ccw construction
  line L61 (18.380184, -65.366371) -> (43.035533, -94.165467) construction
  arc A65 (43.035533, -94.165467) -> (45.41996, -94.667984) centre (44.554817, -92.864785) ccw construction
  arc A66 (45.41996, -94.667984) -> (48.648149, -93.050296) centre (0, 0) ccw construction
  arc A67 (48.648149, -93.050296) -> (49.379523, -88.270396) centre (47.258202, -90.391716) ccw construction
  line L62 (49.379523, -88.270396) -> (46.315494, -85.206367) construction
  arc A68 (46.315494, -73.892659) -> (46.315494, -85.206367) centre (51.972348, -79.549513) ccw construction
  line L63 (46.315494, -73.892659) -> (73.892659, -46.315494) construction
  arc A69 (85.206367, -46.315494) -> (73.892659, -46.315494) centre (79.549513, -51.972348) ccw construction
  line L64 (85.206367, -46.315494) -> (88.270396, -49.379523) construction
  arc A70 (88.270396, -49.379523) -> (93.050296, -48.648149) centre (90.391716, -47.258202) ccw construction
  arc A71 (93.050296, -48.648149) -> (93.050296, 48.648149) centre (0, 0) ccw construction
  arc A72 (93.050296, 48.648149) -> (88.270396, 49.379523) centre (90.391716, 47.258202) ccw construction
  line L65 (88.270396, 49.379523) -> (85.206367, 46.315494) construction
  arc A73 (73.892659, 46.315494) -> (85.206367, 46.315494) centre (79.549513, 51.972348) ccw construction
  line L66 (73.892659, 46.315494) -> (46.315494, 73.892659) construction
  arc A74 (46.315494, 85.206367) -> (46.315494, 73.892659) centre (51.972348, 79.549513) ccw construction
  line L67 (46.315494, 85.206367) -> (49.379523, 88.270396) construction
  arc A75 (49.379523, 88.270396) -> (48.648149, 93.050296) centre (47.258202, 90.391716) ccw construction
  arc A76 (48.648149, 93.050296) -> (-48.648149, 93.050296) centre (0, 0) ccw construction
  arc A77 (-48.648149, 93.050296) -> (-49.379523, 88.270396) centre (-47.258202, 90.391716) ccw construction
  line L68 (-49.379523, 88.270396) -> (-46.315494, 85.206367) construction
  arc A78 (-46.315494, 73.892659) -> (-46.315494, 85.206367) centre (-51.972348, 79.549513) ccw construction
  line L69 (-46.315494, 73.892659) -> (-73.892659, 46.315494) construction
  arc A79 (-85.206367, 46.315494) -> (-73.892659, 46.315494) centre (-79.549513, 51.972348) ccw construction
  line L70 (-85.206367, 46.315494) -> (-88.270396, 49.379523) construction
  circle A80 centre (-37.830213, 79.549513) radius 1.6 construction
  circle A81 centre (-79.549513, 37.830213) radius 1.6 construction
  circle A82 centre (-79.549513, -37.830213) radius 1.6 construction
  circle A83 centre (79.549513, -37.830213) radius 1.6 construction
  circle A84 centre (37.830213, 79.549513) radius 1.6 construction
  circle A85 centre (79.549513, 37.830213) radius 1.6 construction
  circle A86 centre (-20.557843, -60.854564) radius 1.55 construction
  circle A87 centre (20.557843, -60.854564) radius 1.55 construction
  circle A88 centre (37.830213, -79.549513) radius 1.6 construction
  circle A89 centre (-37.830213, -79.549513) radius 1.6 construction
  line L71 (-46.669048, 63.63961) -> (-26.870058, 43.84062) construction
  arc A90 (-26.870058, 41.012193) -> (-26.870058, 43.84062) centre (-28.284271, 42.426407) ccw construction
  line L72 (-26.870058, 41.012193) -> (-41.012193, 26.870058) construction
  arc A91 (-43.84062, 26.870058) -> (-41.012193, 26.870058) centre (-42.426407, 28.284271) ccw construction
  line L73 (-43.84062, 26.870058) -> (-63.63961, 46.669048) construction
  line L74 (-63.63961, 46.669048) -> (-46.669048, 63.63961) construction
  circle A92 centre (0, 0) radius 101 construction
  circle A93 centre (-101, 0) radius 1.6
  circle A94 centre (-101, 0) radius 4
  line L75 (0, 0) -> (0, 40.133514) construction
  line L76 (19.274559, 40.133514) -> (-19.274559, 40.133514) construction
  line L77 (0, 0) -> (-40.133514, 0) construction
  circle A95 centre (101, 0) radius 1.6
  circle A96 centre (101, 0) radius 4
  circle A97 centre (-90.365885, -45.111051) radius 1.6
  line L78 (-46.669048, -63.63961) -> (-63.63961, -46.669048) construction
  line L79 (-55.154329, -55.154329) -> (-33.941125, -33.941125) construction
  circle A98 centre (-45.111051, -90.365885) radius 1.6
  circle A99 centre (-90.365885, 45.111051) radius 1.6
  circle A100 centre (-45.111051, 90.365885) radius 1.6
  circle A101 centre (90.365885, -45.111051) radius 1.6
  circle A102 centre (45.111051, -90.365885) radius 1.6
  circle A103 centre (45.111051, 90.365885) radius 1.6
  circle A104 centre (90.365885, 45.111051) radius 1.6
  dimension "d78" = 202
  dimension "d79" = 3.2
  dimension "d80" = 8
  dimension "d81" = 3.2
  dimension "d84" = 64
  constraints: 13 centre point, 9 symmetric about line, 6 end point, 4 coincident, 4 midpoint, 2 point on circle, 9 other
  measures "d78" diameter of A92
  measures "d79" diameter of A93
  measures "d80" diameter of A94
  measures "d81" diameter of A97
  measures "d84" distance of A97.centre A98.centre
extrude "Выдавливание3" cut sketch "Эскиз3" against normal blind 10 contours A93 | A95 | A97 | A98 | A99 | A100 | A101 | A102 | A103 | A104
extrude "Выдавливание4" add sketch "Эскиз3" against normal blind 2 contours A94 | A96